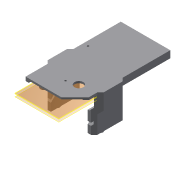
# Autodesk Inventor part: 05_Case_Bottom
Saved by Autodesk Inventor 2016 (Build 200138000, 138)
## iProperties
Created: 2016-11-09
Part Number: 05_Case_Bottom
Material: Generisch
Document SubType Name: Modeling
Designer: Bene
Density: 1 g/cm^3
Appearance: Vorgabe
Author: Bene
Autodesk Inventor part; units mm, degrees
ref_plane "YZ Plane" through (0, 0, 0) normal (1, 0, 0) x (0, 1, 0)
ref_plane "XZ Plane" through (0, 0, 0) normal (0, 1, 0) x (-1, 0, 0)
ref_plane "XY Plane" through (0, 0, 0) normal (0, 0, 1) x (1, 0, 0)
ref_plane "Arbeitsebene1" through (0, 0, 18) normal (0, 0, 1) x (1, 0, 0)
ref_plane "Arbeitsebene2" through (0, 0, 22) normal (0, 0, 1) x (1, 0, 0)
ref_plane "Arbeitsebene4" through (0, 0, 23) normal (0, 0, 1) x (1, 0, 0)
sketch "Skizze1" plane through (0, 0, 23) normal (0, 0, 1) x (1, 0, 0)
  circle A0 centre (13.9714, 39.0775) radius 3.5 construction
  circle A1 centre (-22.5286, -44.9225) radius 3.5 construction
  circle A2 centre (-34.0286, 36.0775) radius 1.5 construction
  circle A3 centre (-4.5286, -28.9225) radius 1.5 construction
  line L0 (5.4714, -49.9225) -> (-36.5286, -49.9225) construction
  line L1 (-36.5286, -49.9225) -> (-36.5286, 73.0775) construction
  line L2 (-36.5286, 73.0775) -> (26.4714, 73.0775) construction
  line L3 (26.4714, 73.0775) -> (26.4714, -28.9225) construction
  line L4 (26.4714, -28.9225) -> (5.4714, -49.9225) construction
  line L5 (-41.5286, -54.9225) -> (7.5424, -54.9225)
  line L6 (7.5424, -54.9225) -> (31.4714, -30.9936)
  line L7 (31.4714, -30.9936) -> (31.4714, 78.0775)
  line L8 (31.4714, 78.0775) -> (-41.5286, 78.0775)
  line L9 (-41.5286, 78.0775) -> (-41.5286, -54.9225)
  dimension "d119" = 5
  constraints: 10 end point, 4 other
  measures "d119" distance between parallel lines of L0 L5
extrude "Extrusion1" add sketch "Skizze1" along normal blind 2
sketch "Skizze2" plane through (0, 0, 23) normal (0, 0, -1) x (-1, 0, 0)
  circle A0 centre (34.0286, 36.0775) radius 3.5
  circle A1 centre (4.5286, -28.9225) radius 3.5
  circle A2 centre (-13.9714, 39.0775) radius 4.5
  circle A3 centre (22.5286, -44.9225) radius 5.5
  circle A4 centre (-13.9714, 39.0775) radius 3.5 construction
  circle A5 centre (22.5286, -44.9225) radius 3.5 construction
  circle A6 centre (34.0286, 36.0775) radius 1.5 construction
  circle A7 centre (4.5286, -28.9225) radius 1.5 construction
  line L0 (-5.4714, -49.9225) -> (36.5286, -49.9225) construction
  line L1 (36.5286, -49.9225) -> (36.5286, 73.0775) construction
  line L2 (36.5286, 73.0775) -> (-26.4714, 73.0775) construction
  line L3 (-26.4714, 73.0775) -> (-26.4714, -28.9225) construction
  line L4 (-26.4714, -28.9225) -> (-5.4714, -49.9225) construction
  point P0 (0, 0)
  dimension "d30" = 54
  constraints: 4 centre point, 2 coincident
ref_plane "Arbeitsebene3" through (-30.2899, -72.9225, 0) normal (0, 0, 1) x (1, 0, 0)
extrude "Extrusion2" add sketch "Skizze2" along normal blind 4
sketch "Skizze3" plane through (0, 0, 25) normal (0, 0, 1) x (1, 0, 0)
  circle A0 centre (13.9714, 39.0775) radius 4.5 construction
  circle A1 centre (-22.5286, -44.9225) radius 5.5 construction
  circle A2 centre (-4.5286, -28.9225) radius 3.5 construction
  circle A3 centre (-34.0286, 36.0775) radius 3.5 construction
  line L0 (-41.5286, -54.9225) -> (7.5424, -54.9225) construction
  line L1 (-41.5286, 78.0775) -> (-41.5286, -54.9225) construction
  line L2 (31.4714, 78.0775) -> (-41.5286, 78.0775) construction
  line L3 (31.4714, -30.9936) -> (31.4714, 78.0775) construction
  line L4 (7.5424, -54.9225) -> (31.4714, -30.9936) construction
  circle A4 centre (11.4714, -23.9225) radius 4.0524 construction
  circle A5 centre (-4.5286, -28.9225) radius 1.5
  circle A6 centre (-34.0286, 36.0775) radius 1.5
  circle A7 centre (11.4714, -23.9225) radius 4.0524 construction
  circle A8 centre (11.4714, -23.9225) radius 4.0524
  point P0 (0, 0)
  dimension "d123" = 2
  dimension "d124" = 2
  constraints: 4 centre point, 2 coincident, 1 concentric
  measures "d123" radial gap between concentric circles of A2 A5
  measures "d124" radial gap between concentric circles of A3 A6
extrude "Extrusion3" cut sketch "Skizze3" against normal through all
sketch "Skizze6" plane through (0, 0, 25) normal (0, 0, 1) x (1, 0, 0)
  line L0 (-41.5286, 78.0775) -> (-41.5286, -54.9225) construction
  circle A0 centre (-34.0286, 36.0775) radius 1.5 construction
  circle A1 centre (-4.5286, -28.9225) radius 1.5 construction
  circle A2 centre (11.4714, -23.9225) radius 4.0524 construction
  line L1 (-41.5286, -54.9225) -> (7.5424, -54.9225) construction
  line L2 (7.5424, -54.9225) -> (31.4714, -30.9936) construction
  line L3 (31.4714, -30.9936) -> (31.4714, 78.0775) construction
  line L4 (31.4714, 78.0775) -> (-41.5286, 78.0775) construction
  line L5 (-41.5286, 78.0775) -> (-41.5286, -54.9225) construction
  line L6 (31.4714, 78.0775) -> (-41.5286, 78.0775) construction
  line L7 (-41.5286, 78.0775) -> (-41.5286, 95.0775) construction
  line L8 (-41.5286, 95.0775) -> (31.4714, 95.0775) construction
  line L9 (31.4714, 95.0775) -> (31.4714, 78.0775) construction
  line L10 (31.4714, 95.0775) -> (31.4714, -30.9936)
  line L11 (31.4714, -30.9936) -> (31.4714, 78.0775) projected
  line L12 (31.4714, -30.9936) -> (7.5424, -54.9225)
  line L13 (-41.5286, -54.9225) -> (7.5424, -54.9225) projected
  line L14 (7.5424, -54.9225) -> (-41.5286, -54.9225)
  line L15 (-41.5286, -54.9225) -> (-41.5286, 95.0775)
  line L16 (-41.5286, 95.0775) -> (31.4714, 95.0775)
  circle A3 centre (11.4714, -23.9225) radius 4.0524 projected
  circle A4 centre (-34.0286, 36.0775) radius 1.5 projected
  circle A5 centre (-4.5286, -28.9225) radius 1.5 projected
  constraints: 18 end point, 3 perpendicular, 2 horizontal, 2 parallel, 1 vertical
extrude "Extrusion6" add sketch "Skizze6" along normal blind 4
sketch "Skizze7" plane through (0, 0, 29) normal (0, 0, 1) x (1, 0, 0)
  line L0 (-41.5286, -54.9225) -> (7.5424, -54.9225) construction
  line L1 (7.5424, -54.9225) -> (31.4714, -30.9936) construction
  line L2 (31.4714, -30.9936) -> (31.4714, 95.0775) construction
  line L3 (31.4714, 95.0775) -> (-41.5286, 95.0775) construction
  line L4 (-41.5286, 95.0775) -> (-41.5286, -54.9225) construction
  line L5 (36.4714, 100.0775) -> (36.4714, -33.0647) construction
  line L6 (36.4714, -33.0647) -> (9.6135, -59.9225) construction
  line L7 (9.6135, -59.9225) -> (-46.5286, -59.9225) construction
  line L8 (-46.5286, -59.9225) -> (-46.5286, 100.0775) construction
  line L9 (-46.5286, 100.0775) -> (36.4714, 100.0775) construction
  line L10 (31.4714, 95.0775) -> (-41.5286, 95.0775) projected
  line L11 (31.4714, 95.0775) -> (36.4714, 95.0775)
  line L12 (36.4714, 95.0775) -> (36.4714, -33.0647)
  line L13 (36.4714, -33.0647) -> (14.6135, -54.9225)
  line L14 (7.5424, -54.9225) -> (31.4714, -30.9936) projected
  line L15 (7.5424, -54.9225) -> (14.6135, -54.9225)
  line L16 (31.4714, -30.9936) -> (31.4714, 95.0775) projected
  line L17 (31.4714, -30.9936) -> (31.4714, 95.0775)
  dimension "d129" = 5
  constraints: 20 end point, 3 perpendicular, 2 point on line, 1 vertical, 4 other
  measures "d129" distance between parallel lines of L2 L5
extrude "Extrusion7" add sketch "Skizze7" against normal up to surface (4 mm away)
sketch "Skizze8" plane through (0, 0, 25) normal (0, 0, -1) x (-1, 0, 0)
  line L0 (-31.4714, 78.0775) -> (41.5286, 78.0775) construction
  line L1 (41.5286, 95.0775) -> (41.5286, 78.0775) construction
  line L2 (-31.4714, -30.9936) -> (-31.4714, 78.0775) construction
  line L3 (-31.4714, 78.0775) -> (41.5286, 78.0775) construction
  line L4 (-36.4714, 95.0775) -> (-28.4714, 95.0775)
  line L5 (-28.4714, 95.0775) -> (-28.4714, 78.0775)
  line L6 (-28.4714, 78.0775) -> (-36.4714, 78.0775)
  line L7 (-36.4714, 78.0775) -> (-36.4714, 95.0775)
  line L8 (-31.4714, 95.0775) -> (41.5286, 95.0775) construction
  line L9 (24.5286, 95.0775) -> (16.5286, 95.0775)
  line L10 (16.5286, 95.0775) -> (16.5286, 78.0775)
  line L11 (16.5286, 78.0775) -> (24.5286, 78.0775)
  line L12 (24.5286, 78.0775) -> (24.5286, 95.0775)
  line L13 (-31.4714, 95.0775) -> (41.5286, 95.0775) projected
  line L14 (-36.4714, 95.0775) -> (-36.4714, -33.0647) projected
  line L15 (-36.4714, -33.0647) -> (-14.6135, -54.9225) projected
  line L16 (-14.6135, -54.9225) -> (-7.5424, -54.9225) projected
  line L17 (-31.4714, -30.9936) -> (-7.5424, -54.9225) projected
  line L18 (-31.4714, 95.0775) -> (-36.4714, 95.0775) projected
  line L19 (-36.4714, 78.0775) -> (-28.4714, 78.0775)
  line L20 (-28.4714, 78.0775) -> (-28.4714, 74.0775)
  line L21 (-28.4714, 74.0775) -> (-36.4714, 74.0775)
  line L22 (-36.4714, 74.0775) -> (-36.4714, 78.0775)
  line L23 (16.5286, 78.0775) -> (24.5286, 78.0775)
  line L24 (24.5286, 78.0775) -> (24.5286, 74.0775)
  line L25 (24.5286, 74.0775) -> (16.5286, 74.0775)
  line L26 (16.5286, 74.0775) -> (16.5286, 78.0775)
  dimension "d126" = 8
  dimension "d127" = 8
  dimension "d128" = 45
  dimension "d225" = 4
  dimension "d226" = 4
  constraints: 32 end point, 8 parallel, 4 horizontal, 4 perpendicular, 3 point on line
  measures "d126" distance of L5.end L6.end
  measures "d127" distance of L11.end L10.end
  measures "d128" distance between parallel lines of L5 L10
  measures "d225" distance of L19.end L20.end
  measures "d226" distance of L23.end L24.end
ref_plane "Arbeitsebene5" through (-15.0286, 71.0775, -46) normal (0, 0, -1) x (0, 1, 0)
extrude "Extrusion8" add sketch "Skizze8" along normal blind 54 contours L12 L11 L10 L9 | L24 L25 L26 L11
sketch "Skizze12" plane through (0, 0, 29) normal (0, 0, 1) x (1, 0, 0)
  line L0 (36.4714, 20.0775) -> (32.077, 20.0775)
  line L1 (26.4714, 16.5537) -> (26.4714, -14.9225)
  line L2 (26.4714, -14.9225) -> (36.4714, -14.9225)
  line L3 (36.4714, -14.9225) -> (36.4714, 20.0775)
  line L4 (-41.5286, -14.9225) -> (-31.5286, -14.9225)
  line L5 (-31.5286, -14.9225) -> (-31.5286, 20.0775)
  line L6 (-31.5286, 20.0775) -> (-41.5286, 20.0775)
  line L7 (-41.5286, 20.0775) -> (-41.5286, -14.9225)
  line L8 (26.4714, 16.5537) -> (33.4714, 16.5537)
  line L9 (33.4714, 16.5537) -> (33.4714, 12.5537)
  line L10 (33.4714, 12.5537) -> (26.4714, 12.5537)
  line L11 (26.4714, 12.5537) -> (26.4714, 16.5537)
  line L12 (-31.5286, 16.5537) -> (-39.0481, 16.5537)
  line L13 (-39.0481, 16.5537) -> (-39.0481, 12.5537)
  line L14 (-39.0481, 12.5537) -> (-31.5286, 12.5537)
  line L15 (-31.5286, 12.5537) -> (-31.5286, 16.5537)
  line L16 (-30.5286, 13.0775) -> (19.4714, 13.0775) construction
  line L17 (-30.5286, 16.0775) -> (-30.5286, 13.0775) construction
  line L18 (19.4714, 16.0775) -> (-30.5286, 16.0775) construction
  line L19 (19.4714, 16.0775) -> (19.4714, 13.0775) construction
  line L20 (33.4714, 16.5537) -> (32.077, 20.0775)
  line L21 (-41.5286, -14.9225) -> (-31.5286, -14.9225)
  line L22 (-31.5286, -14.9225) -> (-31.5286, -24.9225)
  line L23 (-31.5286, -24.9225) -> (-41.5286, -24.9225)
  line L24 (-41.5286, -24.9225) -> (-41.5286, -14.9225)
  line L25 (26.4714, -14.9225) -> (36.4714, -14.9225)
  line L26 (36.4714, -14.9225) -> (36.4714, -24.9225)
  line L27 (36.4714, -24.9225) -> (26.4714, -24.9225)
  line L28 (26.4714, -24.9225) -> (26.4714, -14.9225)
  dimension "d43" = 10
  dimension "d45" = 10
  dimension "d46" = 7
  dimension "d50" = 35
  dimension "d51" = 0
  dimension "d130" = 35
  dimension "d131" = 4
  dimension "d132" = 4
  dimension "d133" = 4
  dimension "d200" = 10
  dimension "d201" = 10
  dimension "d202" = 10
  dimension "d203" = 10
  constraints: 50 end point, 12 parallel, 6 horizontal, 6 perpendicular, 2 point on line
  measures "d43" distance of L2.end L1.end
  measures "d45" distance of L6.end L5.end
  measures "d46" distance of L9.end L10.end
  measures "d50" distance between parallel lines of L4 L6
  measures "d51" distance between parallel lines of L2 L4
  measures "d130" distance between parallel lines of L2 L0
  measures "d131" distance between parallel lines of L6 L18
  measures "d132" distance between parallel lines of L10 L8
  measures "d133" distance between parallel lines of L14 L12
  measures "d200" distance of L22.end L23.end
  measures "d201" distance of L21.end L22.end
  measures "d202" distance of L26.end L27.end
  measures "d203" distance of L25.end L26.end
extrude "Extrusion11" add sketch "Skizze12" against normal up to surface (58 mm away) contours L3 L2 L1 L10 L9 L20 L0 | L26 L27 L28 L2 | L7 L6 L5 L12 L13 L14 L4 | L4 L22 L23 L24
sketch "Skizze15" plane through (-31.5286, -14.9225, -29) normal (1, 0, 0) x (0, 0, -1)
  line L0 (-43.1951, 17.3667) -> (-41.7809, 18.7809) construction
  line L1 (-41.7809, 18.7809) -> (-12.0824, -10.9176) construction
  line L2 (-12.0824, -10.9176) -> (-13.4966, -12.3318) construction
  line L3 (-13.4966, -12.3318) -> (-43.1951, 17.3667) construction
  line L4 (-43.9022, 17.3667) -> (-41.7809, 19.488)
  line L5 (-41.7809, 19.488) -> (-11.3753, -10.9176)
  line L6 (-11.3753, -10.9176) -> (-13.4966, -13.0389)
  line L7 (-13.4966, -13.0389) -> (-43.9022, 17.3667)
  line L8 (-28.8151, 6.5222) -> (-30.9364, 4.4008)
  dimension "d134" = 0.5
  constraints: 10 end point, 2 point on line, 1 perpendicular, 3 other
  measures "d134" distance between parallel lines of L3 L7
ref_plane "Arbeitsebene6" through (-39.5286, -47.0381, -39.7014) normal (-1, 0, 0) x (0, 0, 1)
extrude "Extrusion21" cut sketch "Skizze15" along normal blind 65 and the other way blind 7 contours L8 L5 L6 L7
sketch "Skizze26" plane through (-31.5286, -14.9225, -29) normal (0, 0, -1) x (-1, 0, 0)
  line L0 (7.5194, 27.4762) -> (7.5194, 31.4762) projected
  line L1 (0, 27.4762) -> (7.5194, 27.4762) projected
  line L2 (10, 35) -> (10, -10) projected
  line L3 (0, 35) -> (10, 35) projected
  line L4 (0, 31.4762) -> (0, 35) projected
  line L5 (7.5194, 31.4762) -> (0, 31.4762) projected
  line L6 (-7, 110) -> (-15, 110) projected
  line L7 (-15, 110) -> (-15, 89) projected
  line L8 (-7, 89) -> (-7, 110) projected
  circle A0 centre (-11, 105) radius 3.2 projected
  line L9 (-65, 27.4762) -> (-58, 27.4762) projected
  line L10 (-65, 31.4762) -> (-65, 27.4762) projected
  line L11 (-58, 27.4762) -> (-58, -10) projected
  line L12 (-68, 35) -> (-63.6057, 35) projected
  line L13 (-68, -10) -> (-68, 35) projected
  circle A1 centre (5, 5) radius 4
  circle A2 centre (-63, 5) radius 4
  circle A3 centre (-11, 105) radius 3
  line L14 (-63.6057, 35) -> (-65, 31.4762) projected
  line L15 (-58, -10) -> (-68, -10) projected
  line L16 (0, -10) -> (0, 27.4762) projected
  line L17 (10, -10) -> (0, -10) projected
  line L18 (-15, 89) -> (-7, 89) projected
  point P0 (-31.5286, 14.9225)
  dimension "d142" = 8
  dimension "d143" = 8
  dimension "d144" = 5
  dimension "d149" = 6
  dimension "d152" = 5
  dimension "d153" = 4
  constraints: 3 centre point
  measures "d142" diameter of A1
  measures "d143" diameter of A2
  measures "d144" distance from line of A2.centre L13
  measures "d149" diameter of A3
  measures "d152" distance from line of A3.centre L6
  measures "d153" distance from line of A3.centre L7
extrude "Extrusion22" add sketch "Skizze26" along normal blind 2 contours A1 | A2 | A3
sketch "Skizze27" plane through (0, 0, -29) normal (0, 0, -1) x (-1, 0, 0)
  line L0 (24.5286, 95.0775) -> (16.5286, 95.0775) projected
  line L1 (16.5286, 95.0775) -> (16.5286, 74.0775) projected
  line L2 (24.5286, 74.0775) -> (24.5286, 95.0775) projected
  circle A0 centre (-32.4714, 90.0775) radius 3 projected
  line L3 (-28.4714, 95.0775) -> (-36.4714, 95.0775) projected
  line L4 (-36.4714, 95.0775) -> (-36.4714, 74.0775) projected
  line L5 (-28.4714, 74.0775) -> (-28.4714, 95.0775) projected
  circle A1 centre (36.5286, -9.9225) radius 4 projected
  circle A2 centre (-31.4714, -9.9225) radius 4 projected
  circle A3 centre (-227.2996, 545.8056) radius 1.75
  circle A4 centre (-32.4714, 79.0775) radius 1.75
  circle A5 centre (20.5286, 79.0775) radius 1.75
  line L6 (38.5286, -8.4004) -> (-33.4714, -8.4004) projected
  circle A6 centre (-31.4714, 7.5537) radius 1.75
  line L7 (-33.4714, 12.5537) -> (-26.4714, 12.5537) projected
  circle A7 centre (36.5286, 9.3037) radius 1.75
  circle A8 centre (-32.4714, 79.0775) radius 2.25 projected
  circle A9 centre (20.5286, 79.0775) radius 2.25 projected
  line L8 (-36.4714, 74.0775) -> (-28.4714, 74.0775) projected
  line L9 (16.5286, 74.0775) -> (24.5286, 74.0775) projected
  point P0 (0, 0)
  point P1 (31.5286, -8.4004)
  dimension "d156" = 3.5
  dimension "d157" = 3.5
  dimension "d159" = 3.5
  dimension "d161" = 3.5
  dimension "d162" = 5
  dimension "d163" = 3.5
  dimension "d192" = 4
  dimension "d193" = 4
  dimension "d223" = 0
  dimension "d224" = 0
  constraints: 5 centre point
  measures "d156" diameter of A3
  measures "d157" diameter of A4
  measures "d159" diameter of A5
  measures "d161" diameter of A6
  measures "d162" distance from line of A6.centre L7
  measures "d163" diameter of A7
  measures "d192" distance from line of A5.centre L1
  measures "d193" distance from line of A4.centre L4
  measures "d223" distance of A8.centre A4.centre
  measures "d224" distance of A9.centre A5.centre
extrude "Extrusion23" cut sketch "Skizze27" against normal blind 15 contours A4 | A5 | A6 | A7
sketch "Skizze29" plane through (0, 0, 25) normal (0, 0, -1) x (-1, 0, 0)
  line L0 (-36.4714, 20.0775) -> (-32.077, 20.0775) projected
  line L1 (-31.4714, -30.9936) -> (-31.4714, -24.9225) projected
  line L2 (-36.4714, 95.0775) -> (-36.4714, 20.0775) projected
  line L3 (-36.4714, -33.0647) -> (-14.6135, -54.9225) projected
  line L4 (-14.6135, -54.9225) -> (-7.5424, -54.9225) projected
  line L5 (-31.4714, -30.9936) -> (-7.5424, -54.9225) projected
  line L6 (-33.4714, 12.5537) -> (-31.4714, 12.5537) projected
  line L7 (-32.077, 20.0775) -> (-33.4714, 16.5537) projected
  line L8 (-33.4714, 16.5537) -> (-33.4714, 12.5537) projected
  line L9 (-31.4714, -24.9225) -> (-36.4714, -24.9225) projected
  line L10 (-36.4714, -24.9225) -> (-36.4714, -33.0647) projected
  line L11 (-31.4714, 12.5537) -> (-31.4714, 78.0775) projected
  line L12 (-31.4714, 78.0775) -> (16.5286, 78.0775) projected
  line L13 (16.5286, 78.0775) -> (16.5286, 95.0775) projected
  line L14 (-31.4714, 95.0775) -> (16.5286, 95.0775) projected
  line L15 (-31.4714, 95.0775) -> (-36.4714, 95.0775) projected
  point P0 (0, 0)
extrude "Extrusion25" add sketch "Skizze29" along normal blind 7 contours L2 L15 L14 L13 L12 L11 L6 L8 L7 L0
sketch "Skizze31" plane through (0, 0, 29) normal (0, 0, 1) x (1, 0, 0)
  line L0 (-41.5286, -14.9225) -> (-46.5286, -14.9225)
  line L1 (-46.5286, -14.9225) -> (-46.5286, 20.0775)
  line L2 (-46.5286, 20.0775) -> (-41.5286, 20.0775)
  line L3 (-41.5286, 20.0775) -> (-41.5286, -14.9225)
  line L4 (36.4714, -14.9225) -> (41.4714, -14.9225)
  line L5 (41.4714, -14.9225) -> (41.4714, 20.0775)
  line L6 (41.4714, 20.0775) -> (36.4714, 20.0775)
  line L7 (36.4714, 20.0775) -> (36.4714, -14.9225)
  point P0 (0, 0)
  point P1 (-41.5286, 20.0775)
  point P2 (36.4714, 20.0775)
  dimension "d178" = 5
  dimension "d179" = 5
  constraints: 16 end point, 4 parallel, 2 horizontal, 2 perpendicular, 1 point on line
  measures "d178" distance of L1.end L2.end
  measures "d179" distance of L6.end L5.end
extrude "Extrusion27" add sketch "Skizze31" against normal blind 25
chamfer "Fase6" distance 5 angle 45 12 edges at (-41.5286, 2.5775, 4) (36.4714, 2.5775, 4) (-24.5286, 86.5775, 25) (36.4714, -14.9225, 14.5) (36.4714, -14.9225, 27) (36.4714, -24.9225, -2) (-41.5286, -14.9225, 13.5) (-41.5286, -14.9225, 24) (-41.5286, -14.9225, 27) (-41.5286, -24.9225, -3) (-46.5286, 20.0775, 16.5) (41.4714, 20.0775, 16.5)
sketch "Skizze34" plane through (26.4714, -24.9225, -29) normal (0, -1, 0) x (1, 0, 0)
  line L0 (5, 12.2929) -> (0, 12.2929) construction
  line L1 (0, 12.2929) -> (0, 0) construction
  line L2 (0, 0) -> (5, 0) construction
  line L3 (0, 52) -> (5, 52) construction
  line L4 (0, 52) -> (0, 16.5356) construction
  line L5 (0, 16.5356) -> (5, 16.5356) construction
  line L6 (-58, 12.2929) -> (-63, 12.2929) construction
  line L7 (-63, 16.5356) -> (-58, 16.5356) construction
  line L8 (-58, 52) -> (-58, 16.5356) construction
  line L9 (-63, 52) -> (-58, 52) construction
  line L10 (-63, 0) -> (-58, 0) construction
  line L11 (-58, 12.2929) -> (-58, 0) construction
  line L12 (7.5, 52) -> (-63, 52)
  line L13 (-63, 52) -> (-63, 32)
  line L14 (-63, 32) -> (7.5, 32)
  line L15 (7.5, 32) -> (7.5, 52)
  line L16 (5, 12.2929) -> (5, 0) projected
  line L17 (5, 52) -> (5, 16.5356) projected
  line L18 (-63, 16.5356) -> (-63, 52) projected
  line L19 (-63, 0) -> (-63, 12.2929) projected
  point P0 (-26.4714, 29)
  dimension "d206" = 20
  constraints: 8 end point, 2 parallel, 1 horizontal, 1 perpendicular, 1 point on line
  measures "d206" distance between parallel lines of L12 L14
extrude "Extrusion30" cut sketch "Skizze34" against normal up to surface (45 mm away)
chamfer "Fase7" distance 5 angle 45 3 edges at (33.9714, -1.1725, 3) (-36.5286, 18.3156, 3) (-36.5286, -6.1844, 3)
chamfer "Fase8" distance 5 angle 60 2 edges at (26.4714, 12.5537, -20) (26.4714, 12.5537, -4) measured on face at (26.9714, 12.5537, -4) measured on face at (26.9714, 12.5537, -20)
sketch "Skizze35" plane through (0, 0, 29) normal (0, 0, 1) x (1, 0, 0)
  circle A0 centre (-34.0286, 36.0775) radius 1.5 projected
  circle A1 centre (-4.5286, -28.9225) radius 1.5 projected
  circle A2 centre (11.4714, -23.9225) radius 4.0524 projected
  line L0 (36.4714, 20.0775) -> (41.4714, 15.0775) projected
  line L1 (36.4714, 20.0775) -> (36.4714, 95.0775) projected
  line L2 (36.4714, 95.0775) -> (31.4714, 95.0775) projected
  line L3 (31.4714, 95.0775) -> (-41.5286, 95.0775) projected
  line L4 (-41.5286, 95.0775) -> (-41.5286, 20.0775) projected
  line L5 (-46.5286, 15.0775) -> (-41.5286, 20.0775) projected
  line L6 (-46.5286, 15.0775) -> (-46.5286, -14.9225) projected
  line L7 (-41.5286, -19.9225) -> (-46.5286, -14.9225) projected
  line L8 (-41.5286, -19.9225) -> (-41.5286, -24.9225) projected
  line L9 (-41.5286, -24.9225) -> (-41.5286, -54.9225) projected
  line L10 (-41.5286, -54.9225) -> (7.5424, -54.9225) projected
  line L11 (7.5424, -54.9225) -> (14.6135, -54.9225) projected
  line L12 (14.6135, -54.9225) -> (36.4714, -33.0647) projected
  line L13 (36.4714, -33.0647) -> (36.4714, -24.9225) projected
  line L14 (36.4714, -24.9225) -> (36.4714, -19.9225) projected
  line L15 (41.4714, -14.9225) -> (36.4714, -19.9225) projected
  line L16 (41.4714, -14.9225) -> (41.4714, 15.0775) projected
  circle A3 centre (11.4714, -23.9225) radius 7
  point P0 (0, 0)
  dimension "d213" = 14
  constraints: 1 centre point, 1 coincident
  measures "d213" diameter of A3
extrude "Extrusion31" cut sketch "Skizze35" against normal blind 10 contours A3
sketch "Skizze36" plane through (0, 0, 23) normal (0, 0, -1) x (-1, 0, 0)
  circle A0 centre (-11.4714, -23.9225) radius 7 construction
  circle A1 centre (-13.9714, 39.0775) radius 4.5 construction
  circle A2 centre (34.0286, 36.0775) radius 3.5 construction
  circle A3 centre (22.5286, -44.9225) radius 5.5 construction
  circle A4 centre (4.5286, -28.9225) radius 3.5 construction
  line L0 (36.5286, 12.5537) -> (39.0481, 12.5537) construction
  line L1 (39.0481, 12.5537) -> (39.0481, 16.5537) construction
  line L2 (39.0481, 16.5537) -> (36.5286, 16.5537) construction
  line L3 (36.5286, 16.5537) -> (36.5286, 20.0775) construction
  line L4 (36.5286, 20.0775) -> (41.5286, 20.0775) construction
  line L5 (41.5286, 78.0775) -> (41.5286, 20.0775) construction
  line L6 (27.5286, 78.0775) -> (41.5286, 78.0775) construction
  line L7 (-33.9714, 20.0775) -> (-31.4714, 20.0775) construction
  line L8 (-33.9714, -22.4225) -> (-33.9714, 20.0775) construction
  line L9 (-31.4714, -24.9225) -> (-33.9714, -22.4225) construction
  line L10 (-31.4714, -30.9936) -> (-31.4714, -24.9225) construction
  line L11 (-7.5424, -54.9225) -> (-31.4714, -30.9936) construction
  line L12 (41.5286, -54.9225) -> (-7.5424, -54.9225) construction
  line L13 (41.5286, -19.9225) -> (41.5286, -54.9225) construction
  line L14 (41.5286, -19.9225) -> (36.5286, -24.9225) construction
  line L15 (36.5286, -24.9225) -> (36.5286, 12.5537) construction
  line L16 (29.5286, 78.0775) -> (41.5286, 78.0775) projected
  line L17 (36.5286, 78.0775) -> (-31.4714, 78.0775)
  line L18 (-31.4714, 78.0775) -> (-31.4714, -54.9225)
  line L19 (-31.4714, -54.9225) -> (36.5286, -54.9225)
  circle A5 centre (-13.9714, 39.0775) radius 4.5 projected
  circle A6 centre (-11.4714, -23.9225) radius 7 projected
  circle A7 centre (4.5286, -28.9225) radius 3.5 projected
  circle A8 centre (22.5286, -44.9225) radius 5.5 projected
  circle A9 centre (34.0286, 36.0775) radius 3.5 projected
  circle A10 centre (34.0286, 36.0775) radius 1.5 projected
  arc A11 (36.5286, 41.5318) -> (36.5286, 30.6231) centre (34.0286, 36.0775) ccw
  line L20 (36.5286, -54.9225) -> (36.5286, 30.6231)
  line L21 (36.5286, 33.628) -> (36.5286, 38.5269)
  line L22 (36.5286, 41.5318) -> (36.5286, 78.0775)
  line L23 (36.5286, 12.5537) -> (36.5286, -24.9225) projected
  line L24 (36.5286, -24.9225) -> (41.5286, -19.9225)
  line L25 (41.5286, -54.9225) -> (-7.5424, -54.9225) projected
  line L26 (41.5286, -54.9225) -> (36.5286, -54.9225)
  line L27 (27.5286, 78.0775) -> (27.5286, 74.0775) projected
  line L28 (27.5286, 74.0775) -> (16.5286, 74.0775) projected
  line L29 (16.5286, 74.0775) -> (16.5286, 78.0775) projected
  line L30 (-31.4714, 78.0775) -> (16.5286, 78.0775) projected
  line L31 (-31.4714, 20.0775) -> (-31.4714, 78.0775) projected
  point P0 (0, 0)
  dimension "d30" = 54
  dimension "d218" = 12
  constraints: 16 end point, 4 parallel, 4 point on circle, 2 collinear, 1 centre point, 1 coincident, 1 horizontal, 1 perpendicular, 1 point on line
  measures "d218" diameter of A11
extrude "Extrusion32" cut sketch "Skizze36" against normal blind 3 contours L16 L22 A11 L20 L19 L18 L17 L29 L28 L27 | L27 L28 L29 L17
sketch "Skizze38" plane through (-24.5286, 78.0775, -53) normal (-1, 0, 0) x (0, 0, 1)
  circle A0 centre (40, 6) radius 1.5 projected
  circle A1 centre (58.5, 6) radius 1.5 projected
  line L0 (73, 17) -> (73, -4) projected
  line L1 (73, 17) -> (24, 17) projected
  line L2 (24, -4) -> (24, 17) projected
  circle A2 centre (40, 6) radius 1.5
  circle A3 centre (58.5, 6) radius 1.5
  circle A4 centre (16.4844, 2) radius 1.5
  circle A5 centre (34.961, 2) radius 1.5
  line L3 (73, -4) -> (24, -4) projected
  point P0 (53, -78.0775)
  dimension "d219" = 3
  dimension "d220" = 3
  constraints: 4 centre point, 2 coincident, 2 concentric
  measures "d219" diameter of A4
  measures "d220" diameter of A5
extrude "Extrusion33" cut sketch "Skizze38" against normal through all contours A4 | A5
